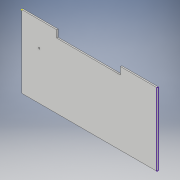
# Autodesk Inventor part: new back support 2
Saved by Autodesk Inventor 2019 (Build 230136000, 136)
## iProperties
Created: 2020-03-01
Part Number: new back support 2
Material: Generic
Document SubType Name: Modeling
Designer: KiranM
Density: 1 g/cm^3
Appearance: Default
Author: KiranM
Autodesk Inventor part; units mm, degrees
ref_plane "YZ Plane" through (0, 0, 0) normal (1, 0, 0) x (0, 1, 0)
ref_plane "XZ Plane" through (0, 0, 0) normal (0, 1, 0) x (-1, 0, 0)
ref_plane "XY Plane" through (0, 0, 0) normal (0, 0, 1) x (1, 0, 0)
sketch "Sketch1" plane through (0, 0, 0) normal (0, 0, 1) x (1, 0, 0)
  line L0 (0, 0) -> (460, 0)
  line L1 (460, 0) -> (460, -250)
  line L2 (460, -250) -> (0, -250)
  line L3 (0, -250) -> (0, 0)
  line L4 (0, 0) -> (120, 0)
  line L5 (120, 0) -> (120, -25)
  line L6 (120, -25) -> (320, -25)
  line L7 (320, -25) -> (340, -25)
  line L8 (340, -25) -> (340, 0)
  line L9 (340, 0) -> (460, 0)
  constraints: 20 end point, 4 perpendicular, 3 point on line, 2 parallel, 1 collinear, 1 horizontal
extrude "Extrusion1" add sketch "Sketch1" along normal blind 5 contours L0 L5 L6 L7 L8 L1 L2 L3
sketch "Sketch2" plane through (0, 0, 5) normal (0, 0, 1) x (1, 0, 0)
  circle A0 centre (60, -85) radius 2.5
  point P0 (0, 0)
  constraints: 1 centre point
extrude "Extrusion2" cut sketch "Sketch2" against normal through all
sketch "Sketch3" plane through (460, -250, 0) normal (1, 0, 0) x (0, 0, -1)
  line L0 (-5, 250) -> (-5, 0) projected
  line L1 (0, 0) -> (-5, 0) projected
  line L2 (-5, 250) -> (0, 250)
  line L3 (0, 250) -> (0, 0)
  line L4 (0, 0) -> (-5, 0)
  line L5 (-5, 0) -> (-5, 250)
  constraints: 8 end point, 2 parallel, 1 horizontal, 1 perpendicular
extrude "Extrusion3" add sketch "Sketch3" along normal blind 5
sketch "Sketch4" plane through (0, 0, 5) normal (0, 0, 1) x (1, 0, 0)
  point P0 (0, 0)
sketch "Sketch5" plane through (465, -250, 0) normal (1, 0, 0) x (0, 0, -1)
  line L0 (0, 250) -> (-5, 250) projected
  line L1 (0, 250) -> (0, 0) projected
  line L2 (-5, 250) -> (0, 250)
  line L3 (0, 250) -> (0, 0)
  line L4 (0, 0) -> (-5, 0)
  line L5 (-5, 0) -> (-5, 250)
  constraints: 8 end point, 2 parallel, 1 horizontal, 1 perpendicular
body "Solid1"
